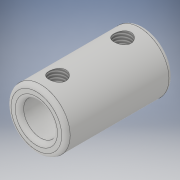
# Autodesk Inventor part: AcopleMotor
Saved by Autodesk Inventor 2019 (Build 230136000, 136)
## iProperties
Created: 2019-05-15
Part Number: AcopleMotor
Material: Generic
Document SubType Name: Modeling
Designer: Iván
Density: 1 g/cm^3
Appearance: Default
Author: Iván
Autodesk Inventor part; units mm, degrees
ref_plane "YZ Plane" through (0, 0, 0) normal (1, 0, 0) x (0, 1, 0)
ref_plane "XY Plane" through (0, 0, 0) normal (0, 0, 1) x (1, 0, 0)
sketch "Sketch1" plane through (0, 0, 0) normal (0, 0, 1) x (1, 0, 0)
  circle A0 centre (0, 0) radius 7
  circle A1 centre (0, 0) radius 4
  dimension "d0" = 14
  dimension "d1" = 8
  constraints: 4 coincident, 2 centre point
  measures "d0" diameter of A0
  measures "d1" diameter of A1
extrude "Extrusion1" add sketch "Sketch1" along normal blind 25.4
fillet "Fillet1" radius 1 2 edges at (-7, 0, 25.4) (-7, 0, 0)
fillet "Fillet2" radius 1 2 edges at (-4, 0, 25.4) (-4, 0, 0)
ref_plane "Work Plane1" through (0, 7, 0) normal (0, 1, 0) x (-1, 0, 0)
sketch "Sketch2" plane through (0, 7, 0) normal (0, 1, 0) x (-1, 0, 0)
  circle A0 centre (0, 5) radius 2
  circle A1 centre (0, 20.4) radius 2
  line L0 (-6, 25.4) -> (6, 25.4) projected
  point P0 (0, 0)
  dimension "d6" = 4
  dimension "d7" = 5
  dimension "d8" = 5
  constraints: 2 centre point, 2 vertical alignment, 1 equal radius
  measures "d6" diameter of A0
  measures "d7" distance of point (0, 0) A0.centre
  measures "d8" distance from line of A1.centre L0
extrude "Extrusion2" cut sketch "Sketch2" against normal up to next
thread "Thread1" size "M4x0.7" class "6H" standard "ANSI Metric M Profile" full length
thread "Thread2" size "M4x0.7" class "6H" standard "ANSI Metric M Profile" full length
equation "\"d8\" = d7"
body "Solid1"
